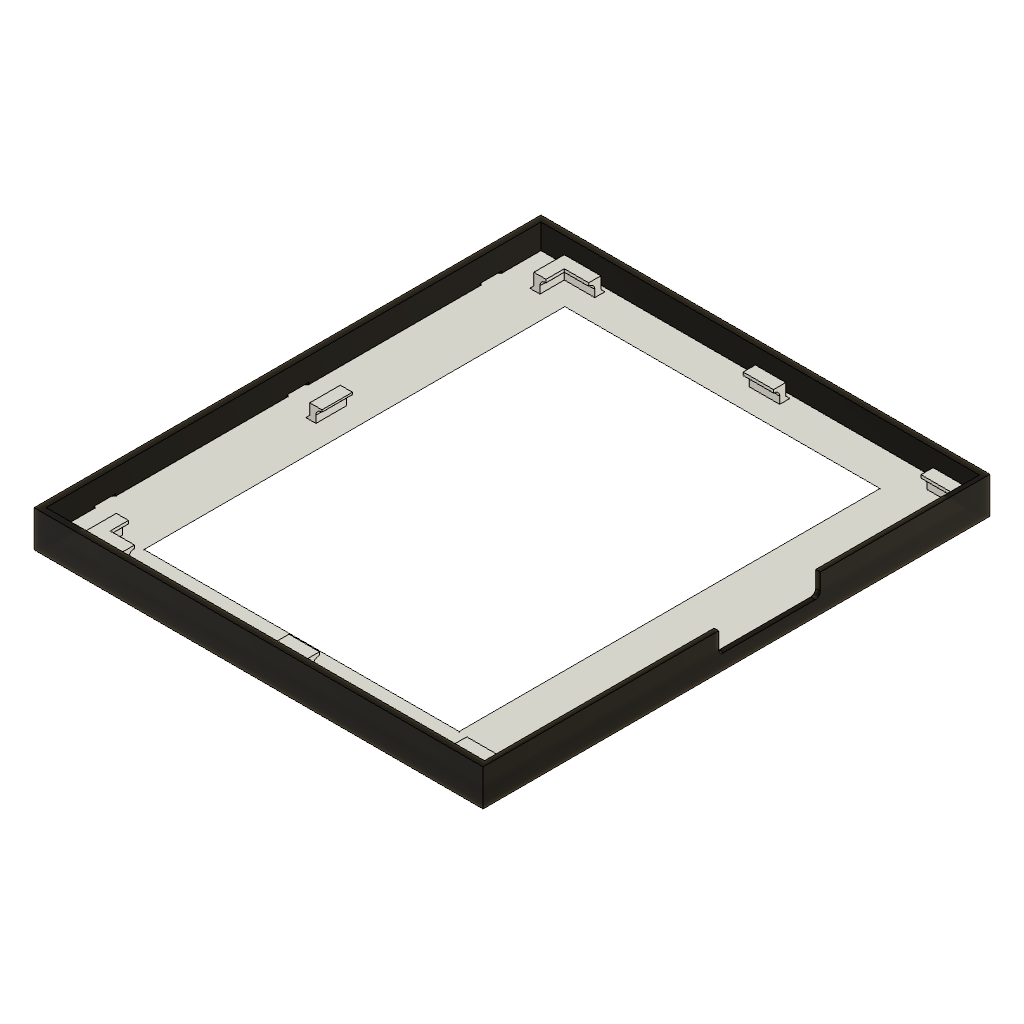
scribe_1 (Autodesk Fusion 360 design; units mm, degrees)
Autodesk Fusion 360 part; units mm, degrees
note: some values were not read from the file. Chosen so that the rebuilt part matches the saved one: which face or edge a step refers to. Set by a fixed rule: which sketch regions a step uses.
sketch "Sketch1" plane through (0, 0, 0) normal (0, 0, 1) x (1, 0, 0)
  line L0 (0, 0) -> (155, 0)
  line L1 (155, 0) -> (155, -207)
  line L2 (155, -207) -> (0, -207)
  line L3 (0, -207) -> (0, 0)
  line L4 (185, -225.25) -> (-30, -225.25)
  line L5 (-30, -225.25) -> (-30, 18.25)
  line L6 (-30, 18.25) -> (185, 18.25)
  line L7 (185, 18.25) -> (185, -225.25)
  line L8 (155, -103.5) -> (0, -103.5) construction
  line L9 (77.5, -103.5) -> (77.5, 0) construction
  line L10 (77.5, -103.5) -> (87, -103.5) construction
  line L11 (185.5, 11.25) -> (-11.5, 11.25)
  line L12 (-11.5, 11.25) -> (-11.5, -218.25)
  line L13 (-11.5, -218.25) -> (185.5, -218.25)
  line L14 (185.5, -218.25) -> (185.5, 11.25)
  line L15 (185.5, 11.25) -> (-11.5, -218.25) construction
  line L16 (-11.5, 11.25) -> (185.5, -218.25) construction
  line L17 (182, 11.25) -> (167, 11.25)
  line L18 (167, 11.25) -> (167, 14.25)
  line L19 (167, 14.25) -> (182, 14.25)
  line L20 (182, 14.25) -> (182, 11.25)
  line L21 (-27, 15.25) -> (182, 15.25)
  line L22 (182, 15.25) -> (182, -222.25)
  line L23 (182, -222.25) -> (-27, -222.25)
  line L24 (-27, -222.25) -> (-27, 15.25)
  line L25 (188, 21.25) -> (188, -228.25)
  line L26 (188, -228.25) -> (-33, -228.25)
  line L27 (-33, -228.25) -> (-33, 21.25)
  line L28 (-33, 21.25) -> (188, 21.25)
  line L29 (94.5, 11.25) -> (79.5, 11.25)
  line L30 (79.5, 11.25) -> (79.5, 14.25)
  line L31 (79.5, 14.25) -> (94.5, 14.25)
  line L32 (94.5, 14.25) -> (94.5, 11.25)
  line L33 (-11.5, 11.25) -> (3.5, 11.25)
  line L34 (3.5, 11.25) -> (3.5, 14.25)
  line L35 (3.5, 14.25) -> (-14.5, 14.25)
  line L36 (-11.5, -96) -> (-14.5, -96)
  line L37 (-14.5, -96) -> (-14.5, -111)
  line L38 (-14.5, -111) -> (-11.5, -111)
  line L39 (-11.5, -111) -> (-11.5, -96)
  line L40 (182, -218.25) -> (167, -218.25)
  line L41 (167, -218.25) -> (167, -221.25)
  line L42 (167, -221.25) -> (182, -221.25)
  line L43 (182, -221.25) -> (182, -218.25)
  line L44 (94.5, -218.25) -> (79.5, -218.25)
  line L45 (79.5, -218.25) -> (79.5, -221.25)
  line L46 (79.5, -221.25) -> (94.5, -221.25)
  line L47 (94.5, -221.25) -> (94.5, -218.25)
  line L48 (3.5, -218.25) -> (-11.5, -218.25)
  line L49 (-11.5, -221.25) -> (3.5, -221.25)
  line L50 (3.5, -221.25) -> (3.5, -218.25)
  line L51 (-11.5, -221.25) -> (-14.5, -221.25)
  line L52 (-14.5, -221.25) -> (-14.5, -206.25)
  line L53 (-14.5, -206.25) -> (-11.5, -206.25)
  line L54 (-11.5, -206.25) -> (-11.5, -218.25)
  line L55 (-14.5, 14.25) -> (-14.5, -0.75)
  line L56 (-14.5, -0.75) -> (-11.5, -0.75)
  line L57 (-11.5, -0.75) -> (-11.5, 11.25)
  line L58 (182, -218.25) -> (167, -218.25)
  line L59 (167, -218.25) -> (167, -215.25)
  line L60 (167, -215.25) -> (182, -215.25)
  line L61 (182, -215.25) -> (182, -218.25)
  line L62 (94.5, -218.25) -> (79.5, -218.25)
  line L63 (79.5, -218.25) -> (79.5, -215.25)
  line L64 (79.5, -215.25) -> (94.5, -215.25)
  line L65 (94.5, -215.25) -> (94.5, -218.25)
  line L66 (3.5, -218.25) -> (-11.5, -218.25)
  line L67 (-8.5, -215.25) -> (3.5, -215.25)
  line L68 (3.5, -215.25) -> (3.5, -218.25)
  line L69 (-11.5, -111) -> (-8.5, -111)
  line L70 (-8.5, -111) -> (-8.5, -96)
  line L71 (-8.5, -96) -> (-11.5, -96)
  line L72 (-11.5, -96) -> (-11.5, -111)
  line L73 (-11.5, -206.25) -> (-8.5, -206.25)
  line L74 (-8.5, -206.25) -> (-8.5, -215.25)
  line L75 (3.5, 11.25) -> (-11.5, 11.25)
  line L76 (-8.5, 8.25) -> (3.5, 8.25)
  line L77 (3.5, 8.25) -> (3.5, 11.25)
  line L78 (-11.5, -0.75) -> (-8.5, -0.75)
  line L79 (-11.5, 11) -> (-11.5, -0.75)
  line L80 (167, 14.25) -> (167, 8.25)
  line L81 (167, 8.25) -> (182, 8.25)
  line L82 (182, 8.25) -> (182, 11.25)
  line L83 (94.5, 11.25) -> (79.5, 11.25)
  line L84 (79.5, 11.25) -> (79.5, 8.25)
  line L85 (79.5, 8.25) -> (94.5, 8.25)
  line L86 (94.5, 8.25) -> (94.5, 11.25)
  line L87 (-8.5, -0.75) -> (-8.5, 8.25)
  point P0 (87, -103.5)
  dimension "d15" = 155
  dimension "d16" = 207
  dimension "d18" = 9.5
  dimension "d19" = 197
  dimension "d20" = 229.5
  dimension "d21" = 15
  dimension "d22" = 3
  dimension "d25" = 3
  dimension "d40" = 15
  dimension "d41" = 15
  dimension "d43" = 3
  dimension "d45" = 3
  dimension "d46" = 15
  dimension "d59" = 15
  dimension "d61" = 15
  dimension "d63" = 3
  dimension "d64" = 3
  dimension "d68" = 3
  dimension "d72" = 15
  dimension "d73" = 3
  dimension "d126" = 18.25
  dimension "d127" = 18.25
  dimension "d129" = 30
  dimension "d130" = 30
  constraint horizontal L0
  constraint vertical L1
  constraint horizontal L2
  constraint vertical L3
  constraint coincident L0.start L3.end
  constraint midpoint L1 L8.start
  constraint midpoint L3 L8.end
  constraint midpoint L8 L9.start
  constraint midpoint L0 L9.end
  constraint perpendicular L9 L10
  constraint horizontal L11
  constraint perpendicular L11 L12
  constraint parallel L11 L13
  constraint parallel L12 L14
  constraint coincident L15 P0
  constraint coincident L16 P0
  constraint coincident P0 L10.end
  constraint horizontal L17
  constraint vertical L18
  constraint horizontal L19
  constraint vertical L20
  constraint coincident L11 L17.start
  constraint horizontal L29
  constraint vertical L30
  constraint horizontal L31
  constraint vertical L32
  constraint coincident L11 L29.start
  constraint horizontal L33
  constraint vertical L34
  constraint horizontal L35
  constraint horizontal L36
  constraint vertical L37
  constraint horizontal L38
  constraint vertical L39
  constraint coincident L12 L36.start
  constraint horizontal L40
  constraint vertical L41
  constraint horizontal L42
  constraint vertical L43
  constraint coincident L13 L40.start
  constraint coincident L22 L40.start
  constraint horizontal L44
  constraint vertical L45
  constraint horizontal L46
  constraint vertical L47
  constraint coincident L13 L44.start
  constraint horizontal L48
  constraint horizontal L49
  constraint vertical L50
  constraint coincident L13 L48.start
  constraint horizontal L51
  constraint vertical L52
  constraint horizontal L53
  constraint vertical L54
  constraint vertical L55
  constraint horizontal L56
  constraint vertical L57
  constraint horizontal L58
  constraint vertical L59
  constraint horizontal L60
  constraint vertical L61
  constraint horizontal L62
  constraint vertical L63
  constraint horizontal L64
  constraint vertical L65
  constraint horizontal L66
  constraint horizontal L67
  constraint vertical L68
  constraint horizontal L69
  constraint vertical L70
  constraint horizontal L71
  constraint vertical L72
  constraint horizontal L73
  constraint vertical L74
  constraint horizontal L75
  constraint horizontal L76
  constraint vertical L77
  constraint horizontal L78
  constraint vertical L87
  constraint vertical L79
  constraint vertical L80
  constraint horizontal L81
  constraint vertical L82
  constraint horizontal L83
  constraint vertical L84
  constraint horizontal L85
  constraint vertical L86
  constraint coincident L20 L17.start
  constraint midpoint L13 L62
  constraint midpoint L11 L29
  constraint equal L53 L73
  constraint coincident L12 L13.start
  constraint midpoint L12 L72
  constraint equal L37 L70
  constraint equal L36 L71
  constraint equal L31 L85
  constraint equal L42 L60
  constraint equal L41 L59
  constraint equal L32 L86
  constraint equal L46 L64
  constraint equal L47 L65
  constraint equal L49 L52
  constraint equal L50 L68
  constraint equal L68 L73
  constraint equal L48 L52
  constraint equal L20 L82
  constraint equal L19 L81
  constraint coincident L19 L18.end
  constraint coincident L22 L17.start
  constraint equal L34 L77
  constraint coincident L11.end L12.start
  constraint equal L77 L78
  constraint equal L56 L78
  constraint equal L55 L75
  constraint coincident L11.end L12
  measures "d15" distance of L0.start L0.end
  measures "d16" distance of L0.start L2.end
  measures "d18" distance of L9.start P0
  measures "d19" distance of L12.end L13.end
  measures "d20" distance of L11.end L12.end
  measures "d21" distance of L17.start L17.end
  measures "d22" distance of L17.start L19.end
  measures "d40" distance of L11.end L33.end
  measures "d41" distance of L36.start L38.end
  measures "d43" distance of L40.start L42.end
  measures "d45" distance of L44.start L46.end
  measures "d46" distance of L48.start L12.end
  measures "d59" distance of L40.start L40.end
  measures "d61" distance of L44.start L44.end
  measures "d63" distance of L48.start L67.end
  measures "d64" distance of L38.end L69.end
  measures "d68" distance of L33.end L76.end
  measures "d72" distance of L29.start L29.end
  measures "d73" distance of L29.start L85.end
  measures "d126" distance of L0 L6
  measures "d127" distance of L2 L4
  measures "d129" distance of L1 L7
  measures "d130" distance of L3 L5
extrude "Extrude4" add sketch "Sketch1" along normal blind 1 contours L4 L5 L6 L7 L11 L13 L20 L21 L22 L23 L24 L43 | L7 L11 L13 L22 L61 L82 | L13 L22 L40 L41 L42 L43 L58 | L13 L22 L40 L58 L59 L60 L61 | L11 L17 L22 L80 L81 L82 | L11 L17 L18 L19 L20 L22 L80 | L11 L12 L13 L18 L19 L21 L22 L23 L24 L30 L31 L32 L34 L35 L36 L37 L38 L41 L42 L45 L46 L47 L49 L50 L51 L52 L53 L55 L56 L80 | L11 L12 L13 L22 L59 L60 L63 L64 L65 L67 L68 L69 L70 L71 L73 L74 L76 L77 L78 L80 L81 L84 L85 L86 L87 | L13 L44 L45 L46 L47 L62 | L13 L44 L62 L63 L64 L65 | L11 L29 L83 L84 L85 L86 | L11 L29 L30 L31 L32 L83 | L12 L13 L48 L49 L50 L51 L52 L53 L54 L66 | L12 L13 L48 L54 L66 L67 L68 L73 L74 | L11 L12 L33 L57 L75 L76 L77 L78 L79 L87 | L11 L12 L33 L34 L35 L55 L56 L57 L75 L79 | L12 L36 L37 L38 L39 L72 | L12 L39 L69 L70 L71 L72 makes body 1
sketch "Sketch2" plane through (154.5, 0, 0) normal (1, 0, 0) x (0, 1, 0)
  line L0 (-122.5, 13) -> (-122.5, 0)
  line L1 (32.5, 0) -> (32.5, 13)
  line L2 (32.5, 13) -> (-122.5, 13)
  line L3 (27.5, 1) -> (-117.5, 1)
  line L4 (-103.5, 0) -> (-103.5, 56.1767)
  line L5 (-103.5, 56.1767) -> (-123.5, 56.1767) construction
  line L6 (-123.5, 56.1767) -> (-83.5, 56.1767)
  line L7 (-83.5, 56.1767) -> (-83.5, 13)
  line L8 (-83.5, 13) -> (-123.5, 13)
  line L9 (-123.5, 13) -> (-123.5, 56.1767)
  line L10 (-122.5, 0) -> (32.5, 0)
  point P0 (-103.5, 0)
  dimension "d31" = 20
  dimension "d32" = 40
  constraint coincident P0 L4.start
  constraint perpendicular L3 L4
  constraint perpendicular L4 L5
  constraint horizontal L6
  constraint vertical L7
  constraint horizontal L8
  constraint vertical L9
  constraint coincident L2 L7.end
  measures "d31" distance of L4.end L5.end
  measures "d32" distance of L5.end L6.end
extrude "Extrude7" add sketch "Sketch1" against normal blind 5 separate body contours L4 L5 L6 L7 L11 L13 L20 L21 L22 L23 L24 L43 | L7 L11 L13 L22 L61 L82 | L7 L11 L13 L14 | L25 L26 L27 L28 makes body 2
extrude "Extrude8" add sketch "Sketch1" along normal blind 13 contours L7 L11 L13 L14 | L25 L26 L27 L28 bodies 2
chamfer "Chamfer1" distance 1 angle 45 4 edges at (155, -103.5, 0) (77.5, 0, 0) (0, -103.5, 0) (77.5, -207, 0) on bodies 1
extrude "Extrude9" add sketch "Sketch1" along normal blind 7.3 from surface at 1 contours L13 L22 L40 L41 L42 L43 L58 | L11 L17 L18 L19 L20 L22 L80 | L13 L44 L45 L46 L47 L62 | L11 L29 L30 L31 L32 L83 | L12 L13 L48 L49 L50 L51 L52 L53 L54 L66 | L11 L12 L33 L34 L35 L55 L56 L57 L75 L79 | L12 L36 L37 L38 L39 L72 bodies 1
chamfer "Chamfer2" distance 2 angle 45 9 edges at (174.5, 14.25, 1) (87, 14.25, 1) (-5.5, 14.25, 1) (-14.5, 6.75, 1) (-14.5, -103.5, 1) (-14.5, -213.75, 1) (-5.5, -221.25, 1) (87, -221.25, 1) (174.5, -221.25, 1) on bodies 1
extrude "Extrude10" cut sketch "Sketch2" against normal blind 5 contours L2 L4 L6 L8 L9 | L2 L4 L6 L7 L8 bodies 2
fillet "Fillet1" [no effect]
extrude "Extrude11" add sketch "Sketch1" against normal blind 1 from surface at 8.3 contours L13 L22 L40 L58 L59 L60 L61 | L11 L17 L22 L80 L81 L82 | L13 L44 L62 L63 L64 L65 | L11 L29 L83 L84 L85 L86 | L12 L13 L48 L54 L66 L67 L68 L73 L74 | L11 L12 L33 L57 L75 L76 L77 L78 L79 L87 | L12 L39 L69 L70 L71 L72 bodies 1
extrude "Extrude12" add 6 faces at (177, -218.25, 8.3) (84.5, -220.25, 8.3) (-12.5, -214.25, 8.3) (-6.5, 12.25, 8.3) (89.5, 11.25, 8.3) (177, 10.25, 8.3) along direction (0, 0, 1) blind 0.5 on bodies 1 bodies 1
move_face "OffsetFaces3" offset -0.2 4 faces at (41.6667, 18.25, 0.3333) (185, -62.9167, 0.3333) (113.3333, -225.25, 0.3333) (-30, -144.0833, 0.3333) on bodies 1
sketch "Sketch3" plane through (0, -225.25, 0) normal (0, 1, 0) x (-1, 0, 0)
  line L0 (-185, 0) -> (30, 0)
  line L1 (30, 0) -> (30, 13)
  line L2 (30, 13) -> (-185, 13)
  line L3 (-185, 13) -> (-185, 0)
  line L4 (-125, 1) -> (-62, 1)
  line L5 (-62, 1) -> (-62, -9)
  line L6 (-62, -9) -> (-125, -9)
  line L7 (-125, -9) -> (-125, 1)
  line L8 (29.8, 1) -> (-184.8, 1)
  line L9 (-125, 1) -> (-115, 1)
  line L10 (-115, 1) -> (-115, 3)
  line L11 (-115, 3) -> (-125, 3)
  line L12 (-125, 3) -> (-125, 1)
  dimension "d80" = 10
  dimension "d81" = 2
  constraint horizontal L4
  constraint vertical L5
  constraint horizontal L6
  constraint vertical L7
  constraint coincident L4.start L8
  constraint horizontal L9
  constraint vertical L10
  constraint horizontal L11
  constraint vertical L12
  measures "d80" distance of L4.start L9.end
  measures "d81" distance of L4.start L11.end
sketch "Sketch4" plane through (0, 0, 1) normal (0, 0, 1) x (-1, 0, 0)
  line L0 (-184.8, 225.05) -> (-184.8, -18.05)
  line L1 (-184.8, -18.05) -> (29.8, -18.05)
  line L2 (29.8, 225.05) -> (-184.8, 225.05)
  line L3 (-155, 0) -> (-155, 207)
  line L4 (30, 103.5) -> (-184.8, 103.5) construction
  line L5 (10, -18.05) -> (0, -18.05)
  line L6 (0, -18.05) -> (0, -19.55)
  line L7 (0, -19.55) -> (10, -19.55)
  line L8 (10, -19.55) -> (10, -18.05)
  line L9 (-164.8, -18.05) -> (-154.8, -18.05)
  line L10 (-154.8, -18.05) -> (-154.8, -19.55)
  line L11 (-154.8, -19.55) -> (-164.8, -19.55)
  line L12 (-164.8, -19.55) -> (-164.8, -18.05)
  line L13 (10, -19.55) -> (11.5, -18.05)
  line L14 (10, -19.55) -> (9.6213, -19.55) construction
  line L15 (0, -19.55) -> (-1.5, -18.05)
  line L16 (-154.8, -19.55) -> (-153.3, -18.05)
  line L17 (-164.8, -19.55) -> (-166.3, -18.05)
  line L18 (10, 226.55) -> (10, 225.05)
  line L19 (10, 226.55) -> (11.5, 225.05)
  line L20 (0, 226.55) -> (10, 226.55)
  line L21 (10, 225.05) -> (0, 225.05)
  line L22 (0, 225.05) -> (0, 226.55)
  line L23 (0, 226.55) -> (-1.5, 225.05)
  line L24 (-154.8, 226.55) -> (-153.3, 225.05)
  line L25 (-154.8, 225.05) -> (-154.8, 226.55)
  line L26 (-164.8, 225.05) -> (-154.8, 225.05)
  line L27 (-154.8, 226.55) -> (-164.8, 226.55)
  line L28 (-164.8, 226.55) -> (-164.8, 225.05)
  line L29 (-164.8, 226.55) -> (-166.3, 225.05)
  line L30 (30, 225.25) -> (30, -18.25)
  line L31 (-167, 223.25) -> (-167, 218.25)
  line L32 (-167, 218.25) -> (-182, 218.25)
  line L33 (-182, 218.25) -> (-182, 223.25)
  line L34 (-182, 223.25) -> (-167, 223.25)
  line L35 (-182, -16.25) -> (-182, -11.25)
  line L36 (-182, -11.25) -> (-167, -11.25)
  line L37 (-167, -11.25) -> (-167, -16.25)
  line L38 (-167, -16.25) -> (-182, -16.25)
  line L39 (-79.5, 223.25) -> (-79.5, 218.25)
  line L40 (-79.5, 218.25) -> (-94.5, 218.25)
  line L41 (-94.5, 218.25) -> (-94.5, 223.25)
  line L42 (-94.5, 223.25) -> (-79.5, 223.25)
  line L43 (-94.5, -16.25) -> (-94.5, -11.25)
  line L44 (-94.5, -11.25) -> (-79.5, -11.25)
  line L45 (-79.5, -11.25) -> (-79.5, -16.25)
  line L46 (-79.5, -16.25) -> (-94.5, -16.25)
  line L47 (29.8, -18.05) -> (29.8, 225.05)
  line L48 (-155, 207) -> (0, 207)
  line L49 (0, 207) -> (0, 0)
  line L50 (0, 0) -> (-155, 0)
  line L51 (-3.5, 218.25) -> (-3.5, 223.25)
  line L52 (-3.5, 223.25) -> (16.5, 223.25)
  line L53 (16.5, 223.25) -> (16.5, 206.25)
  line L54 (16.5, 206.25) -> (11.5, 206.25)
  line L55 (11.5, 206.25) -> (11.5, 218.25)
  line L56 (11.5, 218.25) -> (-3.5, 218.25)
  line L57 (11.5, 0.75) -> (16.5, 0.75)
  line L58 (16.5, 0.75) -> (16.5, -16.25)
  line L59 (16.5, -16.25) -> (-3.5, -16.25)
  line L60 (-3.5, -16.25) -> (-3.5, -11.25)
  line L61 (-3.5, -11.25) -> (11.5, -11.25)
  line L62 (11.5, -11.25) -> (11.5, 0.75)
  line L63 (16.5, 96) -> (11.5, 96)
  line L64 (11.5, 96) -> (11.5, 111)
  line L65 (11.5, 111) -> (16.5, 111)
  line L66 (16.5, 111) -> (16.5, 96)
  circle A0 centre (-77.4, 103.5) radius 4.36
  line L67 (31.3, 192.8283) -> (29.8, 191.2254)
  line L68 (31.3, 200.05) -> (31.3, 192.8283)
  line L69 (31.3, 192.8283) -> (29.8, 192.8265)
  line L70 (31.3, 200.05) -> (29.8, 201.4238)
  line L71 (29.8, 200.05) -> (31.3, 200.05)
  line L72 (29.8, 191.2254) -> (29.8, 201.4238)
  line L73 (31.3, 105.05) -> (29.8, 106.4238)
  line L74 (29.8, 105.05) -> (31.3, 105.05)
  line L75 (29.8, 96.2254) -> (29.8, 106.4238)
  line L76 (31.3, 105.05) -> (31.3, 97.8283)
  line L77 (31.3, 97.8283) -> (29.8, 96.2254)
  line L78 (31.3, 97.8283) -> (29.8, 97.8265)
  line L79 (31.3, 10.05) -> (29.8, 11.4238)
  line L80 (29.8, 10.05) -> (31.3, 10.05)
  line L81 (29.8, 1.2254) -> (29.8, 11.4238)
  line L82 (31.3, 10.05) -> (31.3, 2.8283)
  line L83 (31.3, 2.8283) -> (29.8, 1.2254)
  line L84 (31.3, 2.8283) -> (29.8, 2.8265)
  line L85 (-77.875, 227.8) -> (-77.875, -20.8) construction
  line L86 (-187.05, 10.05) -> (-187.05, 2.8283)
  line L87 (-187.05, 2.8283) -> (-185.55, 1.2254)
  line L88 (-187.05, 2.8283) -> (-185.55, 2.8265)
  line L89 (-185.55, 1.2254) -> (-185.55, 11.4238)
  line L90 (-187.05, 10.05) -> (-185.55, 11.4238)
  line L91 (-185.55, 10.05) -> (-187.05, 10.05)
  line L92 (-187.05, 97.8283) -> (-185.55, 97.8265)
  line L93 (-187.05, 97.8283) -> (-185.55, 96.2254)
  line L94 (-187.05, 105.05) -> (-187.05, 97.8283)
  line L95 (-185.55, 96.2254) -> (-185.55, 106.4238)
  line L96 (-187.05, 105.05) -> (-185.55, 106.4238)
  line L97 (-185.55, 105.05) -> (-187.05, 105.05)
  line L98 (-187.05, 200.05) -> (-185.55, 201.4238)
  line L99 (-185.55, 200.05) -> (-187.05, 200.05)
  line L100 (-187.05, 200.05) -> (-187.05, 192.8283)
  line L101 (-187.05, 192.8283) -> (-185.55, 192.8265)
  line L102 (-187.05, 192.8283) -> (-185.55, 191.2254)
  line L103 (-185.55, 191.2254) -> (-185.55, 201.4238)
  line L104 (-184.8, -18.05) -> (-184.8, 225.05)
  dimension "d84" = 10
  dimension "d85" = 1.5
  dimension "d86" = 10
  dimension "d87" = 1.5
  dimension "d88" = 45
  dimension "d121" = 20
  dimension "d122" = 20
  dimension "d131" = 1.5
  dimension "d132" = 25
  dimension "d137" = 0
  dimension "d139" = 106.925
  constraint midpoint L0 L4.end
  constraint horizontal L5
  constraint vertical L6
  constraint horizontal L7
  constraint vertical L8
  constraint coincident L1 L5.start
  constraint horizontal L9
  constraint vertical L10
  constraint horizontal L11
  constraint vertical L12
  constraint coincident L1 L9.start
  constraint horizontal L14
  constraint coincident L1 L13.end
  constraint coincident L1 L15.end
  constraint perpendicular L13 L15
  constraint coincident L1 L16.end
  constraint perpendicular L15 L16
  constraint coincident L1 L17.end
  constraint perpendicular L16 L17
  constraint symmetric L4 L5.start L18.end
  constraint symmetric L4 L5.end L21.end
  constraint symmetric L4 L6.end L20.start
  constraint symmetric L4 L7.end L18.start
  constraint symmetric L4 L9.start L26.start
  constraint symmetric L4 L9.end L25.start
  constraint symmetric L4 L10.end L24.start
  constraint symmetric L4 L11.end L27.end
  constraint symmetric L4 L13.end L19.end
  constraint symmetric L4 L15.end L23.end
  constraint symmetric L4 L16.end L24.end
  constraint symmetric L4 L17.end L29.end
  constraint midpoint L4.start L30
  constraint midpoint L4 A0.centre
  constraint perpendicular L71 L72
  constraint coincident L69.end L72
  constraint coincident L71.start L72
  constraint coincident L47 L69.end
  constraint vertical L68
  constraint symmetric L67.start L85 L100.end
  constraint symmetric L69.end L85 L101.end
  constraint symmetric L67.end L85 L102.end
  constraint symmetric L68.start L85 L98.start
  constraint symmetric L71.start L85 L99.start
  constraint symmetric L70.end L85 L98.end
  constraint symmetric L73.start L85 L94.start
  constraint symmetric L73.end L85 L95.end
  constraint symmetric L74.start L85 L97.start
  constraint symmetric L75.start L85 L93.end
  constraint symmetric L76.end L85 L92.start
  constraint symmetric L78.end L85 L92.end
  constraint symmetric L79.start L85 L86.start
  constraint symmetric L79.end L85 L89.end
  constraint symmetric L80.start L85 L91.start
  constraint symmetric L81.start L85 L87.end
  constraint symmetric L82.end L85 L86.end
  constraint symmetric L84.end L85 L88.end
  measures "d84" distance of L5.start L5.end
  measures "d85" distance of L5.start L7.end
  measures "d86" distance of L9.start L9.end
  measures "d87" distance of L9.start L11.end
  measures "d88" angle of L13 L14
  measures "d121" distance of L8 L30
  measures "d122" distance of L0 L12
  measures "d131" distance of L68 L72
  measures "d132" distance of L2 L71
  measures "d139" distance of L85 L104
fillet "Fillet2" radius 2.75 9 edges at (87, 11.25, 7.3) (174.5, 11.25, 7.3) (-4, 11.25, 7.3) (-11.5, 5.25, 7.3) (-11.5, -103.5, 7.3) (-4, -218.25, 7.3) (-11.5, -212.25, 7.3) (87, -218.25, 7.3) (174.5, -218.25, 7.3) on bodies 1
extrude "Extrude13" add 1 faces at (184.8, -62.9833, 0.6667) along direction (1, 0, 0) blind 0.75 on bodies 1 bodies 1
extrude "Extrude14" cut 1 faces at (185, -62.9167, 4.3333) along direction (1, 0, 0) blind 0.75 on bodies 2 bodies 2
extrude "horizontal_lips" [suppressed]
extrude "vertical_lips" add sketch "Sketch4" against normal blind 1 contours L30 L47 L70 L71 L72 | L30 L47 L81 L83 L84 | L30 L47 L69 L71 L72 | L30 L70 L71 | L30 L47 L80 L81 L84 | L30 L83 L84 | L30 L47 L67 L69 L72 | L30 L68 L69 L71 | L30 L47 L79 L80 L81 | L30 L80 L82 L84 | L30 L67 L69 | L30 L79 L80 | L30 L47 L73 L74 L75 | L30 L47 L75 L77 L78 | L30 L47 L74 L75 L78 | L30 L73 L74 | L30 L77 L78 | L30 L74 L76 L78 | L86 L88 L89 L91 | L89 L90 L91 | L87 L88 L89 | L92 L94 L95 L97 | L92 L93 L95 | L95 L96 L97 | L98 L99 L103 | L99 L100 L101 L103 | L101 L102 L103 bodies 1
chamfer "Chamfer3" [suppressed]
chamfer "Chamfer7" distance 0.3 angle 45 12 edges at (-31.3, -6.4391, 1) (-31.3, -6.4391, 0) (-31.3, -101.4391, 1) (-31.3, -101.4391, 0) (-31.3, -196.4391, 1) (-31.3, -196.4391, 0) (187.05, -196.4391, 0) (187.05, -196.4391, 1) (187.05, -101.4391, 1) (187.05, -101.4391, 0) (187.05, -6.4391, 1) (187.05, -6.4391, 0) on bodies 1
combine "Combine2" operation cut target body 2 tool bodies 1 keep tools
move_face "OffsetFaces4" [suppressed]
move_face "OffsetFaces5" offset -0.3 24 faces at (-30.3333, -96.7953, 0.3333) (-31.3, -102.6428, 0.5667) (-30.3333, -100.0625, 1) (-30.3333, -105.9353, 0.3333) (-31.3, -195.2355, 0.4333) (-30.3333, -200.9353, 0.3333) (-30.3333, -195.0625, 1) (-30.6667, -192.1515, 0.3333) (-31.3, -5.2355, 0.4333) (-30.3333, -5.0625, 1) (-30.6667, -10.63, 0.3333) (-30.6667, -2.1515, 0.3333) (186.0833, -1.7953, 0.6667) (187.05, -5.2355, 0.5667) (186.0833, -10.9353, 0.6667) (186.0833, -5.0625, 1) (187.05, -102.6428, 0.4333) (186.0833, -100.0625, 1) (186.4167, -105.63, 0.6667) (186.4167, -97.1515, 0.6667) (187.05, -197.6428, 0.5667) (186.0833, -195.0625, 1) (186.4167, -192.1515, 0.3333) (186.0833, -200.9353, 0.3333) on bodies 2
chamfer "Chamfer4" [suppressed]
chamfer "Chamfer5" distance 3 distance2 5 4 edges at (182, -103.5, -5) (77.5, 15.25, -5) (77.5, -222.25, -5) (-27, -103.5, -5) measured on face at (-31, -143.0833, -5) measured on face at (-31, -143.0833, -5) measured on face at (-31, -143.0833, -5) measured on face at (-31, -143.0833, -5) on bodies 2
chamfer "Chamfer8" distance 0.5 angle 45 6 edges at (185.75, -196.3237, 1.3) (185.75, -101.3237, 1.3) (185.75, -6.3237, 1.3) (-30, -6.3237, 1.3) (-30, -101.3237, 1.3) (-30, -196.3237, 1.3) on bodies 2
sketch "Sketch5" plane through (188, 0, 0) normal (1, 0, 0) x (0, 1, 0)
  line L0 (-228.25, 13) -> (-228.25, -5)
  line L1 (-228.25, -5) -> (21.25, -5)
  line L2 (21.25, -5) -> (21.25, 13)
  line L3 (21.25, 13) -> (-228.25, 13)
  line L4 (-112.2904, 13) -> (-62.2904, 13)
  line L5 (-112.2904, 13) -> (-62.2904, 13)
  line L6 (-62.2904, 13) -> (-62.2904, 2.5)
  line L7 (-62.2904, 2.5) -> (-112.2904, 2.5)
  line L8 (-112.2904, 2.5) -> (-112.2904, 13)
  point P0 (-87.2904, 13)
  dimension "d147" = 50
  dimension "d148" = 10.5
  constraint midpoint L4 P0
  constraint coincident L3 P0
  constraint parallel L3 L4
  constraint horizontal L5
  constraint vertical L6
  constraint horizontal L7
  constraint vertical L8
  constraint coincident L4.end L6
  measures "d147" distance of L4.start L4.end
  measures "d148" distance of L4.start L7.end
extrude "Extrude17" cut sketch "Sketch5" against normal blind 2.25 contours L3 L4 L5 L6 L7 L8 bodies 2
fillet "Fillet3" radius 2.5 2 edges at (186.875, -112.2904, 2.5) (186.875, -62.2904, 2.5) on bodies 2
equation "d15 = screen_height"
equation "d16 = screen_width"
equation "d18 = ( screen_bott_padding - screen_top_padding ) / 2"
equation "d19 = kindle_height"
equation "d20 = kindle_width"
equation "d21 = holder_lengh"
equation "d22 = holder_width"
equation "d25 = bezel_width"
equation "d26 = -( bezel_width )"
equation "d40 = holder_lengh"
equation "d41 = holder_lengh"
equation "d43 = holder_width"
equation "d45 = holder_width"
equation "d46 = holder_lengh"
equation "d52 = holder_height"
equation "d59 = holder_lengh"
equation "d61 = holder_lengh"
equation "d63 = holder_width"
equation "d64 = holder_width"
equation "d68 = holder_width"
equation "d72 = holder_lengh"
equation "d73 = holder_width"
equation "bezel_width = 3 mm" comment "3.00"
equation "screen_width = 207 mm" comment "207.00"
equation "screen_height = 155 mm" comment "155.00"
equation "kindle_height = 197 mm" comment "196.50"
equation "kindle_width = 229.5 mm" comment "229.00"
equation "screen_bott_padding = 30 mm" comment "30.00"
equation "screen_top_padding = 11 mm" comment "11.00"
equation "holder_lengh = 15 mm" comment "15.00"
equation "holder_width = 3 mm" comment "3.00"
equation "screen_side_padding = ( kindle_width - screen_width ) / 2" comment "11.00"
equation "carton_bezel_padding_horizontal = 7 mm" comment "10.00"
equation "d126 = screen_side_padding + carton_bezel_padding_horizontal"
equation "d127 = screen_side_padding + carton_bezel_padding_horizontal"
equation "carton_bezel_padding_vertical = screen_bott_padding" comment "30.00"
equation "d129 = carton_bezel_padding_vertical"
equation "d130 = carton_bezel_padding_vertical"
equation "vertical_locks_padding = 25 mm"
equation "vertical_locks_position = screen_height + ( carton_bezel_padding_vertical * 2 ) - vertical_locks_padding"
equation "d138 = -vertical_locks_position"
equation "d139 = 107.30 mm - ( ( 0.75 / 2 ) * 1 mm )"
equation "holder_height = 7.3 mm"
